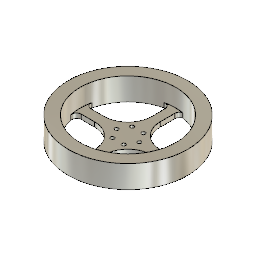
ReactionWheel V2 (Autodesk Fusion 360 design; units mm, degrees)
Autodesk Fusion 360 part; units mm, degrees
note: some values were not read from the file. Set by a fixed rule: which sketch regions a step uses.
cylinder "CylinderPrimitive1" add diameter 100 height 19 placed x (1, 0, 0) y (0, 1, 0) z (0, 0, 1) at (0, 0, 0)
sketch "Esquisse5" plane through (0, 0, 19) normal (0, 0, 1) x (-1, 0, 0)
  circle A0 centre (0, 0) radius 50
  circle A1 centre (0, 0) radius 9.5
  circle A2 centre (-9.5, 0) radius 0.445
  circle A3 centre (4.75, 8.2272) radius 0.445
  circle A4 centre (-4.75, 8.2272) radius 0.445
  circle A5 centre (9.5, 0) radius 0.445
  circle A6 centre (4.75, -8.2272) radius 0.445
  circle A7 centre (-4.75, -8.2272) radius 0.445
  circle A8 centre (0, 0) radius 40
  line L0 (24, 4) -> (35.0999, 4)
  line L1 (35.0999, -4) -> (24, -4)
  line L2 (-4, 24) -> (-4, 35.3488)
  line L3 (4, 35.0999) -> (4, 24)
  arc A9 (4, 24) -> (24, 4) centre (24, 24) ccw
  line L4 (-24, 4) -> (-35.3735, 4)
  line L5 (-35.7211, -3.5) -> (-23.5, -3.5)
  line L6 (-3.5, -23.5) -> (-3.5, -35.7211)
  line L7 (4, -35.0999) -> (4, -24)
  arc A10 (24, -4) -> (4, -24) centre (24, -24) ccw
  arc A11 (-3.5, -23.5) -> (-23.5, -3.5) centre (-23.5, -23.5) ccw
  arc A12 (-24, 4) -> (-4, 24) centre (-24, 24) ccw
  arc A13 (8.8889, -38.9998) -> (38.9998, -8.8889) centre (0, 0) ccw
  arc A14 (4, -35.0999) -> (8.8889, -38.9998) centre (8, -35.0999) ccw
  arc A15 (-8.3219, -39.6358) -> (-3.5, -35.7211) centre (-7.5, -35.7211) ccw
  arc A16 (-35.7211, -3.5) -> (-39.6358, -8.3219) centre (-35.7211, -7.5) ccw
  arc A17 (-8.9237, 39.2407) -> (-39.2645, 8.9272) centre (0.5204, -0.5528) ccw
  arc A18 (38.9998, 8.8889) -> (8.8889, 38.9998) centre (0, 0) ccw
  arc A19 (-39.2645, 8.9272) -> (-35.3735, 4) centre (-35.3735, 8) ccw
  arc A20 (-4, 35.3488) -> (-8.9237, 39.2407) centre (-8, 35.3488) ccw
  arc A21 (8.8889, 38.9998) -> (4, 35.0999) centre (8, 35.0999) ccw
  arc A22 (35.0999, 4) -> (38.9998, 8.8889) centre (35.0999, 8) ccw
  arc A23 (38.9998, -8.8889) -> (35.0999, -4) centre (35.0999, -8) ccw
  point P0 (-4.75, -8.2272)
  point P1 (4.75, -8.2272)
  point P2 (9.5, 0)
  point P3 (4.75, 8.2272)
  point P4 (-4.75, 8.2272)
  point P5 (28, 0)
  point P6 (0, 28)
  point P7 (-28, 0)
  point P8 (0, -28)
  dimension "d13" = 19
  dimension "d14" = 0.89
  dimension "d17" = 0.89
  dimension "d18" = 0.89
  dimension "d19" = 0.89
  dimension "d20" = 0.89
  dimension "d21" = 0.89
  dimension "d31" = 80
  dimension "d35" = 20
  dimension "d38" = 20
  dimension "d39" = 20
  dimension "d40" = 20
  dimension "d41" = 4
  dimension "d42" = 4
  dimension "d43" = 4
  dimension "d44" = 4
  dimension "d45" = 4
  dimension "d46" = 4
  dimension "d47" = 4
  dimension "d48" = 4
  constraint coincident A1 A2.centre
  constraint coincident P3 A3.centre
  constraint coincident P4 A4.centre
  constraint coincident P2 A5.centre
  constraint coincident P1 A6.centre
  constraint coincident P0 A7.centre
  constraint coincident A0.centre A1.centre
  constraint horizontal L0
  constraint parallel L0 L1
  constraint parallel L2 L3
  constraint tangent L0 A9
  constraint tangent L3 A9
  constraint horizontal L4
  constraint parallel L4 L5
  constraint parallel L6 L7
  constraint tangent L1 A10
  constraint tangent L7 A10
  constraint tangent L6 A11
  constraint tangent L5 A11
  constraint tangent L4 A12
  constraint tangent L2 A12
  constraint tangent L7 A14
  constraint tangent A13 A14
  constraint tangent L6 A15
  constraint tangent L5 A16
  constraint tangent L4 A19
  constraint tangent A17 A19
  constraint tangent L2 A20
  constraint tangent A17 A20
  constraint tangent A18 A21
  constraint tangent L3 A21
  constraint tangent A18 A22
  constraint tangent L0 A22
  constraint tangent A13 A23
  constraint tangent L1 A23
  measures "d13" diameter of A1
  measures "d14" diameter of A2
  measures "d17" diameter of A3
  measures "d18" diameter of A4
  measures "d19" diameter of A5
  measures "d20" diameter of A6
  measures "d21" diameter of A7
  measures "d31" diameter of A8
  measures "d35" radius of A9
  measures "d38" radius of A10
  measures "d39" radius of A11
  measures "d40" radius of A12
  measures "d41" radius of A14
  measures "d42" radius of A15
  measures "d43" radius of A16
  measures "d44" radius of A19
  measures "d45" radius of A20
  measures "d46" radius of A21
  measures "d47" radius of A22
  measures "d48" radius of A23
extrude "Extrusion4" cut sketch "Esquisse5" against normal blind 35 contours A8 L0 L3 A9 A18 A21 A22 | A8 L1 L7 A10 A13 A14 A23 | A8 L2 L4 A12 A19 A20 | A8 L5 L6 A11 A15 A16
extrude "Extrusion5" cut sketch "Esquisse5" against normal blind 15 contours A1 A5 | A1 A5 | A1 A2 A3 A4 A5 A6 A7 | A1 A3 | A1 A3 | A1 A6 | A1 A6 | A1 A4 | A1 A4 | A1 A7 | A1 A7 | A1 A2 | A1 A2 | A8 L0 L1 L2 L3 A9 L4 L5 L6 L7 A10 A11 A12 A14 A15 A16 A19 A20 A21 A22 A23
hole "Perçage2" at (4.75, 8.2272, 19) at (9.5, 0, 19) at (-4.75, -8.2272, 19) at (-9.5, 0, 19) at (-4.75, 8.2272, 19) at (4.75, -8.2272, 19) direction (0, 0, -1) diameter 3 depth 33 tip angle 180
